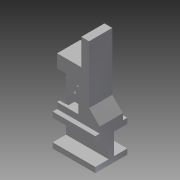
# Autodesk Inventor part: mod_gripper_flat
Saved by Autodesk Inventor 2015 (Build 190159000, 159)
## iProperties
Created: 2014-11-17
Part Number: mod_gripper_flat
Material: Steel, High Strength Low Alloy
Document SubType Name: Modeling
Designer: R.HOLESKO
Manufacturer: Standard
Standards Organization: Custom
Density: 1 g/cm^3
Appearance: Steel
Author: R.HOLESKO
Autodesk Inventor part; units mm, degrees
ref_plane "YZ Plane" through (0, 0, 0) normal (1, 0, 0) x (0, 1, 0)
ref_plane "XZ Plane" through (0, 0, 0) normal (0, 1, 0) x (-1, 0, 0)
ref_plane "XY Plane" through (0, 0, 0) normal (0, 0, 1) x (1, 0, 0)
sketch "Sketch1" plane through (0, 0, 0) normal (0, 0, 1) x (1, 0, 0)
  line L0 (-9.525, 0) -> (9.525, 0)
  line L1 (9.525, 0) -> (9.525, 44.45)
  line L2 (9.525, 44.45) -> (5.715, 44.45)
  line L3 (5.715, 44.45) -> (4.891, 28.7274)
  line L4 (4.891, 28.7274) -> (-9.525, 28.7274)
  line L5 (-9.525, 28.7274) -> (-9.525, 0)
  point P0 (0, 0)
  point P1 (0, 0)
  dimension "d0" = 44.45
  dimension "d1" = 15.24
  dimension "d2" = 15.7226
  dimension "d3" = 19.05
  dimension "d14" = 93
  constraints: 12 end point, 3 horizontal, 2 vertical, 1 coincident, 1 midpoint
  measures "d0" distance of L0.end L1.end
  measures "d1" horizontal distance of L2.end L4.end
  measures "d2" vertical distance of L2.end L4.end
  measures "d3" distance between parallel lines of L1 L5
  measures "d14" angle of L3 L4
extrude "Extrusion1" add sketch "Sketch1" along normal mid plane 15.7226
sketch "Sketch2" plane through (0, 0, 0) normal (1, 0, 0) x (0, 1, 0)
  line L0 (-19.05, 9.525) -> (-19.05, -9.525)
  line L1 (-19.05, -9.525) -> (-15.875, -9.525)
  line L2 (-15.875, -9.525) -> (-15.875, -1.5875)
  line L3 (-15.875, -1.5875) -> (-3.175, -1.5875)
  line L4 (-3.175, -1.5875) -> (-3.175, -9.525)
  line L5 (-3.175, -9.525) -> (0, -9.525)
  line L6 (0, -9.525) -> (0, 9.525)
  line L7 (0, 9.525) -> (-3.175, 9.525)
  line L8 (-3.175, 9.525) -> (-3.175, 1.5875)
  line L9 (-3.175, 1.5875) -> (-15.875, 1.5875)
  line L10 (-15.875, 1.5875) -> (-15.875, 9.525)
  line L11 (-15.875, 9.525) -> (-19.05, 9.525)
  line L12 (0, -7.8613) -> (0, 7.8613) projected
  point P0 (0, 0)
  point P1 (0, 0)
  dimension "d6" = 19.05
  dimension "d7" = 19.05
  dimension "d8" = 3.175
  dimension "d9" = 3.175
  constraints: 24 end point, 6 equal length, 6 horizontal, 6 vertical, 2 midpoint
  measures "d6" distance of L5.end L6.end
  measures "d7" distance of L6.end L0.start
  measures "d8" distance of L4.end L5.end
  measures "d9" distance between parallel lines of L3 L9
extrude "Extrusion2" add sketch "Sketch2" along normal mid plane 19.05
sketch "Sketch6" plane through (0, 0, 7.8613) normal (0, 0, 1) x (1, 0, 0)
  line L0 (4.891, 28.7274) -> (9.525, 28.7274)
  line L1 (9.525, 28.7274) -> (9.525, 44.45)
  line L2 (9.525, 44.45) -> (4.891, 44.45)
  line L3 (4.891, 44.45) -> (4.891, 28.7274)
  point P0 (0, 0)
  constraints: 8 end point, 2 parallel, 1 horizontal, 1 perpendicular
extrude "Extrusion3" add sketch "Sketch6" against normal blind 15.7226
sketch "Sketch9" plane through (0, 0, 7.8613) normal (0, 0, 1) x (1, 0, 0)
  line L0 (4.891, 44.45) -> (4.891, 28.7274) projected
  line L1 (-9.525, 28.7274) -> (-9.525, 0) projected
  line L2 (4.891, 28.7274) -> (-2.729, 28.7274)
  line L3 (4.891, 28.7274) -> (-9.525, 28.7274) projected
  line L4 (-9.525, 28.7274) -> (-9.525, 26.7462)
  line L5 (-9.525, 26.7462) -> (-2.729, 28.7274)
  point P0 (0, 0)
  dimension "d22" = 14.416
  dimension "d23" = 7.62
  dimension "d24" = 1.9812
  constraints: 6 end point, 2 point on line
  measures "d22" distance between parallel lines of L0 L1
  measures "d23" distance of L0.end L2.end
  measures "d24" distance of L1.start L4.end
extrude "Extrusion5" cut sketch "Sketch9" against normal blind 25.4
fillet "Fillet2" radius 5.08 1 edges at (-2.729, 28.7274, 0)
sketch "Sketch10" plane through (-9.525, -15.875, 1.5875) normal (0, 0, 1) x (1, 0, 0)
  circle A0 centre (9.525, 6.35) radius 0.635
  line L0 (0, 0) -> (0, 12.7) projected
  line L1 (19.05, -3.175) -> (0, -3.175) projected
  point P0 (9.525, 15.875)
  dimension "d28" = 9.525
  dimension "d29" = 9.525
  dimension "d30" = 1.27
  constraints: 1 centre point
  measures "d28" distance from line of L0 A0.centre
  measures "d29" distance from line of L1 A0.centre
  measures "d30" diameter of A0
extrude "Extrusion6" cut sketch "Sketch10" against normal blind 25.4
sketch "Sketch12" plane through (-9.525, -15.875, -1.5875) normal (-1, 0, 0) x (0, 0, 1)
  line L0 (-6.2738, 60.325) -> (-6.2738, 15.875) projected
  line L1 (9.4488, 42.6212) -> (9.4488, 15.875) projected
  line L2 (-6.2738, 36.7601) -> (9.4488, 36.7601)
  line L3 (9.4488, 36.7601) -> (9.4488, 19.5053)
  line L4 (9.4488, 19.5053) -> (-6.2738, 19.5053)
  line L5 (-6.2738, 19.5053) -> (-6.2738, 36.7601)
  point P0 (1.5875, 15.875)
  constraints: 8 end point, 2 parallel, 2 point on line, 1 horizontal, 1 perpendicular
extrude "Extrusion7" cut sketch "Sketch12" against normal blind 12.7
sketch "Sketch13" plane through (3.175, -15.875, -1.5875) normal (-1, 0, 0) x (0, 0, 1)
  line L0 (0, 12.7) -> (0, 36.7601)
  line L1 (-6.2738, 36.7601) -> (9.4488, 36.7601) projected
  line L2 (0, 12.7) -> (0, 0) projected
  line L3 (3.175, 12.7) -> (3.175, 36.7601)
  line L4 (3.175, 0) -> (3.175, 12.7) projected
  line L5 (9.4488, 19.5053) -> (-6.2738, 19.5053) projected
  line L6 (0, 36.7601) -> (3.175, 36.7601)
  line L7 (3.175, 36.7601) -> (3.175, 19.5053)
  line L8 (3.175, 19.5053) -> (0, 19.5053)
  line L9 (0, 19.5053) -> (0, 36.7601)
  point P0 (1.5875, 15.875)
  constraints: 12 end point, 4 point on line, 2 collinear, 2 parallel, 1 horizontal, 1 perpendicular
extrude "Extrusion8" add sketch "Sketch13" along normal blind 12.7
sketch "Sketch15" plane through (3.175, 3.6303, 1.5875) normal (0, 0, 1) x (1, 0, 0)
  circle A0 centre (-7.62, 5.0254) radius 0.635
  line L0 (-12.7, 0) -> (-12.7, 17.2548) projected
  circle A1 centre (-5.715, 9.4248) radius 0.635
  circle A2 centre (-5.08, 14.5048) radius 0.635
  point P0 (-3.175, -3.6303)
  dimension "d40" = 5.08
  dimension "d41" = 1.27
  dimension "d42" = 1.27
  dimension "d45" = 1.27
  dimension "d46" = 6.985
  dimension "d47" = 7.62
  constraints: 3 centre point
  measures "d40" distance from line of L0 A0.centre
  measures "d41" diameter of A0
  measures "d42" diameter of A1
  measures "d45" diameter of A2
  measures "d46" distance from line of L0 A1.centre
  measures "d47" distance from line of L0 A2.centre
extrude "Extrusion9" cut sketch "Sketch15" against normal blind 12.7
sketch "Sketch17" plane through (-9.525, -15.875, -1.5875) normal (-1, 0, 0) x (0, 0, 1)
  line L0 (-7.9375, 15.875) -> (11.1125, 15.875)
  line L1 (0, 19.5053) -> (-3.81, 19.5053)
  line L2 (-3.81, 19.5053) -> (-3.81, 15.875)
  line L3 (-3.81, 15.875) -> (0, 15.875)
  line L4 (0, 15.875) -> (0, 19.5053)
  line L5 (3.175, 19.5053) -> (6.985, 19.5053)
  line L6 (6.985, 19.5053) -> (6.985, 15.875)
  line L7 (6.985, 15.875) -> (3.175, 15.875)
  line L8 (3.175, 15.875) -> (3.175, 19.5053)
  point P0 (1.5875, 15.875)
  dimension "d51" = 3.81
  dimension "d52" = 3.81
  constraints: 18 end point, 4 parallel, 3 horizontal, 2 perpendicular, 2 point on line
  measures "d51" distance of L1.start L1.end
  measures "d52" distance of L5.start L5.end
extrude "Extrusion10" cut sketch "Sketch17" against normal blind 5.08
sketch "Sketch18" plane through (9.525, 44.45, 7.8613) normal (1, 0, 0) x (0, 0, -1)
  line L0 (-1.6637, -63.5) -> (-1.6637, -60.325)
  line L1 (-1.6637, -60.325) -> (6.2738, -60.325)
  line L2 (6.2738, -60.325) -> (-1.6637, -60.325) projected
  line L3 (6.2738, -60.325) -> (6.2738, -47.625)
  line L4 (6.2738, -47.625) -> (-1.6637, -47.625)
  line L5 (-1.6637, -47.625) -> (-1.6637, -44.45)
  line L6 (-1.6637, -44.45) -> (-1.6637, -47.625) projected
  line L7 (-1.6637, -44.45) -> (0, -44.45)
  line L8 (0, -44.45) -> (0, -40.8197)
  line L9 (0, -44.45) -> (0, 0) projected
  line L10 (15.7226, 0) -> (15.7226, -44.45) projected
  line L11 (15.7226, -41.3057) -> (15.7226, -44.45)
  line L12 (17.3863, -44.45) -> (15.7226, -44.45) projected
  line L13 (15.7226, -44.45) -> (17.3863, -44.45)
  line L14 (17.3863, -44.45) -> (17.3863, -47.625)
  line L15 (17.3863, -47.625) -> (17.3863, -44.45) projected
  line L16 (17.3863, -47.625) -> (9.4488, -47.625)
  line L17 (9.4488, -47.625) -> (9.4488, -60.325)
  line L18 (17.3863, -60.325) -> (9.4488, -60.325) projected
  line L19 (9.4488, -60.325) -> (17.3863, -60.325)
  line L20 (17.3863, -63.5) -> (17.3863, -60.325) projected
  line L21 (17.3863, -60.325) -> (17.3863, -63.5)
  line L22 (17.3863, -63.5) -> (-1.6637, -63.5)
  line L23 (-1.6637, -63.5) -> (17.3863, -63.5) projected
  line L24 (0, -40.8197) -> (15.7226, -40.8197)
  line L25 (9.4488, -40.8197) -> (15.7226, -40.8197) projected
  line L26 (15.7226, -40.8197) -> (15.7226, -44.45)
  point P0 (7.8613, -44.45)
  constraints: 34 end point, 10 perpendicular, 5 collinear, 3 point on line, 1 vertical
extrude "Extrusion11" add sketch "Sketch18" along normal blind 6.35
chamfer "Chamfer1" distance 6.35 angle 45 1 edges at (9.525, 3.6303, 0)
sketch "Sketch19" plane through (-9.525, -15.875, -1.5875) normal (0, 0, -1) x (-1, 0, 0)
  circle A0 centre (-9.525, 6.35) radius 0.762
  circle A1 centre (-9.525, 6.35) radius 0.635 projected
  point P0 (-9.525, 15.875)
  dimension "d60" = 0
  dimension "d61" = 0
  dimension "d62" = 1.524
  constraints: 1 centre point
  measures "d60" distance of A1.centre A0.centre
  measures "d61" distance of A1.centre A0.centre
  measures "d62" diameter of A0
extrude "Extrusion12" cut sketch "Sketch19" against normal blind 6.35
sketch "Sketch20" plane through (3.175, 3.6303, -1.5875) normal (0, 0, -1) x (-1, 0, 0)
  circle A0 centre (5.08, 14.5048) radius 0.762
  circle A1 centre (5.08, 14.5048) radius 0.635 projected
  circle A2 centre (5.715, 9.4248) radius 0.762
  circle A3 centre (5.715, 9.4248) radius 0.635 projected
  circle A4 centre (7.62, 5.0254) radius 0.762
  circle A5 centre (7.62, 5.0254) radius 0.635 projected
  point P0 (3.175, -3.6303)
  dimension "d65" = 0
  dimension "d66" = 0
  dimension "d67" = 1.524
  dimension "d68" = 0
  dimension "d69" = 0
  dimension "d70" = 1.524
  dimension "d71" = 0
  dimension "d72" = 0
  dimension "d73" = 1.524
  constraints: 3 centre point
  measures "d65" distance of A1.centre A0.centre
  measures "d66" distance of A0.centre A1.centre
  measures "d67" diameter of A0
  measures "d68" distance of A2.centre A3.centre
  measures "d69" distance of A2.centre A3.centre
  measures "d70" diameter of A2
  measures "d71" distance of A5.centre A4.centre
  measures "d72" distance of A5.centre A4.centre
  measures "d73" diameter of A4
extrude "Extrusion13" cut sketch "Sketch20" against normal blind 6.35
sketch "Sketch25" plane through (-9.525, -15.875, -1.5875) normal (-1, 0, 0) x (0, 0, 1)
  line L0 (9.4488, 19.5053) -> (9.4488, 15.875) projected
  line L1 (-6.2738, 15.875) -> (-6.2738, 19.5053) projected
  line L2 (-6.2738, 15.875) -> (-5.3086, 15.875)
  line L3 (-5.3086, 15.875) -> (-5.3086, 64.7795)
  line L4 (-5.3086, 64.7795) -> (-6.2738, 64.7795)
  line L5 (-6.2738, 64.7795) -> (-6.2738, 15.875)
  line L6 (9.4488, 15.875) -> (8.4836, 15.875)
  line L7 (8.4836, 15.875) -> (8.4836, 64.7795)
  line L8 (8.4836, 64.7795) -> (9.4488, 64.7795)
  line L9 (9.4488, 64.7795) -> (9.4488, 15.875)
  point P0 (1.5875, 15.875)
  dimension "d87" = 15.7226
  dimension "d88" = 0.9652
  dimension "d89" = 0.9652
  constraints: 16 end point, 4 parallel, 2 horizontal, 2 perpendicular
  measures "d87" distance between parallel lines of L0 L1
  measures "d88" distance of L3.end L4.end
  measures "d89" distance of L7.end L8.end
extrude "Extrusion16" cut sketch "Sketch25" against normal blind 38.1
sketch "Sketch30" plane through (-9.525, 20.8851, 6.8961) normal (0, 0, 1) x (1, 0, 0)
  line L0 (0, 5.8611) -> (0, 0) projected
  line L1 (14.416, 7.8423) -> (7.5214, 7.8423) projected
  line L2 (0, 2.9305) -> (8.832, 2.9305)
  line L3 (8.832, 2.9305) -> (8.832, 7.8423)
  line L4 (8.832, 7.8423) -> (0, 7.8423)
  line L5 (0, 7.8423) -> (0, 2.9305)
  point P0 (9.525, -20.8851)
  constraints: 8 end point, 2 parallel, 1 horizontal, 1 midpoint, 1 perpendicular, 1 point on line
extrude "Extrusion17" add sketch "Sketch30" against normal blind 13.7922
body "Solid1"
